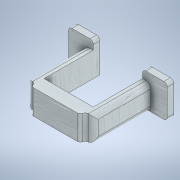
# Autodesk Inventor part: podstawa 01-3
Saved by Autodesk Inventor 2021 (Build 250183000, 183)
## iProperties
Created: 2021-11-05
Part Number: podstawa 01-3
Material: Generic
Document SubType Name: Modeling
Designer: Łukasz
Density: 1 g/cm^3
Appearance: Wood - Painted White
Author: Łukasz
Autodesk Inventor part; units mm, degrees
ref_plane "YZ Plane" through (0, 0, 0) normal (1, 0, 0) x (0, 1, 0)
ref_plane "XZ Plane" through (0, 0, 0) normal (0, 1, 0) x (-1, 0, 0)
ref_plane "XY Plane" through (0, 0, 0) normal (0, 0, 1) x (1, 0, 0)
sketch "Sketch1" plane through (0, 0, 0) normal (0, 0, 1) x (1, 0, 0)
  line L0 (0, 0) -> (40, 0)
  line L1 (40, 0) -> (40, -15)
  line L2 (40, -15) -> (0, -15)
  line L3 (0, -15) -> (0, 0)
  dimension "d0" = 40
  dimension "d1" = 15
  constraints: 8 end point, 2 parallel, 1 horizontal, 1 perpendicular
  measures "d0" distance of L1.end L2.end
  measures "d1" distance of L0.end L1.end
extrude "Extrusion1" add sketch "Sketch1" along normal blind 5
sketch "Sketch2" plane through (0, 0, 5) normal (0, 0, 1) x (1, 0, 0)
  line L0 (40, 0) -> (0, 0) projected
  line L1 (5, 0) -> (35, 0)
  line L2 (35, 0) -> (35, -15)
  line L3 (35, -15) -> (5, -15)
  line L4 (5, -15) -> (5, 0)
  line L5 (0, 0) -> (0, -15) projected
  dimension "d4" = 30
  dimension "d5" = 15
  dimension "d6" = 5
  constraints: 8 end point, 2 parallel, 1 horizontal, 1 perpendicular, 1 point on line
  measures "d4" distance of L2.end L3.end
  measures "d5" distance of L1.end L2.end
  measures "d6" distance between parallel lines of L5 L4
extrude "Extrusion2" add sketch "Sketch2" along normal blind 3
fillet "Fillet1" radius 2 4 edges at (35, -7.5, 5) (35, -7.5, 8) (5, -7.5, 5) (5, -7.5, 8)
sketch "Sketch3" plane through (0, 0, 0) normal (0, 0, -1) x (-1, 0, 0)
  line L0 (0, 0) -> (0, -15) projected
  line L1 (-40, 0) -> (0, 0) projected
  line L2 (0, -15) -> (-5, -15)
  line L3 (-5, -15) -> (-5, 0)
  line L4 (-5, 0) -> (0, 0)
  line L5 (0, 0) -> (0, -15)
  line L6 (-40, -15) -> (-40, 0) projected
  line L7 (0, -15) -> (-40, -15) projected
  line L8 (-40, 0) -> (-35, 0)
  line L9 (-35, 0) -> (-35, -15)
  line L10 (-35, -15) -> (-40, -15)
  line L11 (-40, -15) -> (-40, 0)
  dimension "d10" = 5
  dimension "d11" = 5
  constraints: 16 end point, 4 parallel, 2 horizontal, 2 perpendicular, 2 point on line
  measures "d10" distance of L3.end L4.end
  measures "d11" distance of L9.end L10.end
extrude "Extrusion3" add sketch "Sketch3" along normal blind 34 contours L0 L2 L3 L1 | L9 L7 L6 L1
sketch "Sketch4" plane through (0, 0, -34) normal (0, 0, -1) x (-1, 0, 0)
  line L0 (-35, 0) -> (-35, -15) projected
  line L1 (-35, -15) -> (-50, -15)
  line L2 (-50, -15) -> (-50, 5)
  line L3 (-50, 5) -> (-35, 5)
  line L4 (-35, 5) -> (-35, -15)
  line L5 (-5, -15) -> (-35, -15) projected
  line L6 (-5, -15) -> (10, -15)
  line L7 (10, -15) -> (10, 5)
  line L8 (10, 5) -> (-5, 5)
  line L9 (-5, 5) -> (-5, -15)
  point P0 (-4.9365, 0)
  dimension "d18" = 15
  dimension "d19" = 20
  dimension "d20" = 15
  constraints: 16 end point, 4 parallel, 2 horizontal, 2 perpendicular, 1 point on line
  measures "d18" distance of L2.end L3.end
  measures "d19" distance of L1.end L2.end
  measures "d20" distance of L8.end L7.end
extrude "Extrusion4" add sketch "Sketch4" against normal blind 4
fillet "Fillet2" radius 3 6 edges at (0, 0, -12.5) (0, -7.5, 5) (0, -15, -12.5) (40, -15, -12.5) (40, -7.5, 5) (40, 0, -12.5)
fillet "Fillet3" radius 2 6 edges at (-10, 5, -32) (5, 5, -32) (-10, -15, -32) (35, 5, -32) (50, 5, -32) (50, -15, -32)
body "Solid1"
